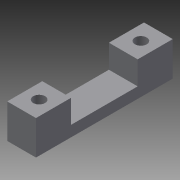
# Autodesk Inventor part: Pump clamp MM0312
Saved by Autodesk Inventor 2013 SP2 (Build 170200200, 200)
## iProperties
Created: 2015-07-10
Part Number: Pump clamp MM0312
Material: Generic
Document SubType Name: Modeling
Designer: kthorn
Density: 1 g/cm^3
Author: kthorn
Autodesk Inventor part; units mm, degrees
ref_plane "YZ Plane" through (0, 0, 0) normal (1, 0, 0) x (0, 1, 0)
ref_plane "XZ Plane" through (0, 0, 0) normal (0, 1, 0) x (-1, 0, 0)
ref_plane "XY Plane" through (0, 0, 0) normal (0, 0, 1) x (1, 0, 0)
sketch "Sketch1" plane through (0, 0, 0) normal (0, 0, 1) x (1, 0, 0)
  line L0 (-44.4426, 24.9959) -> (-36.4426, 24.9959)
  line L1 (-36.4426, 24.9959) -> (-36.4426, -13.0041)
  line L2 (-36.4426, -13.0041) -> (-44.4426, -13.0041)
  line L3 (-44.4426, -13.0041) -> (-44.4426, 24.9959)
  point P0 (0, 0)
  dimension "d0" = 38
  dimension "d2" = 8
  constraints: 8 end point, 2 parallel, 1 horizontal, 1 perpendicular
  measures "d0" distance of L0.end L1.end
  measures "d2" distance of L0.start L0.end
extrude "Extrusion1" add sketch "Sketch1" along normal blind 3
sketch "Sketch2" plane through (0, 0, 3) normal (0, 0, 1) x (1, 0, 0)
  line L0 (-44.4426, 24.9959) -> (-44.4426, -13.0041) construction
  line L1 (-44.4426, -13.0041) -> (-36.4426, -13.0041) projected
  line L2 (-36.4426, -13.0041) -> (-36.4426, 24.9959) projected
  line L3 (-44.4426, 24.9959) -> (-36.4426, 24.9959)
  line L4 (-36.4426, 24.9959) -> (-36.4426, 15.2459)
  line L5 (-36.4426, 15.2459) -> (-44.4426, 15.2459)
  line L6 (-44.4426, 15.2459) -> (-44.4426, 24.9959)
  line L7 (-36.4426, -13.0041) -> (-44.4426, -13.0041)
  line L8 (-44.4426, -13.0041) -> (-44.4426, -3.2541)
  line L9 (-44.4426, -3.2541) -> (-36.4426, -3.2541)
  line L10 (-36.4426, -3.2541) -> (-36.4426, -13.0041)
  point P0 (0, 0)
  dimension "d5" = 9.75
  dimension "d7" = 9.75
  constraints: 16 end point, 4 parallel, 2 horizontal, 2 perpendicular, 2 point on line
  measures "d5" distance of L3.end L4.end
  measures "d7" distance between parallel lines of L1 L9
extrude "Extrusion2" add sketch "Sketch2" along normal blind 6.5
sketch "Sketch3" plane through (0, 0, 9.5) normal (0, 0, 1) x (1, 0, 0)
  line L0 (-36.4426, -13.0041) -> (-36.4426, -3.2541) projected
  line L1 (-36.4426, -3.2541) -> (-44.4426, -3.2541) projected
  line L2 (-44.4426, -3.2541) -> (-44.4426, -13.0041) projected
  line L3 (-44.4426, -13.0041) -> (-36.4426, -13.0041) projected
  line L4 (-36.4426, 24.9959) -> (-44.4426, 15.2459) construction
  line L5 (-36.4426, -3.2541) -> (-44.4426, -13.0041) construction
  circle A0 centre (-40.4426, 20.1209) radius 1.65
  circle A1 centre (-40.4426, -8.1291) radius 1.65
  point P0 (0, 0)
  dimension "d10" = 3.3
  constraints: 4 end point, 2 centre point, 2 midpoint, 1 equal radius, 1 parallel
  measures "d10" diameter of A0
extrude "Extrusion3" cut sketch "Sketch3" against normal through all contours A0 | A1
body "Solid1"
